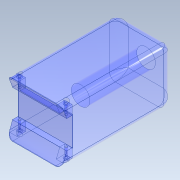
# Autodesk Inventor part: shank_front_v2
Saved by Autodesk Inventor 2020 (Build 240168000, 168)
## iProperties
Created: 2021-01-30
Part Number: shank_front_v2
Material: Generic
Document SubType Name: Modeling
Designer: DELL
Density: 1 g/cm^3
Appearance: Clear - Blue
Mass: 1058.53 g
Surface Area: 891.515 cm^2
Volume: 1058.53 cm^3
Author: DELL
Autodesk Inventor part; units mm, degrees
ref_plane "YZ Plane" through (0, 0, 0) normal (1, 0, 0) x (0, 1, 0)
ref_plane "XY Plane" through (0, 0, 0) normal (0, 0, 1) x (1, 0, 0)
ref_plane "UCS1: YZ Plane" through (0, 0, 0) normal (1, 0, 0) x (0, 1, 0)
sketch "Sketch16" plane through (0, 0, 0) normal (1, 0, 0) x (0, 1, 0)
  circle A0 centre (0, 0) radius 56
  line L0 (0, -212.6874) -> (0, 100.7812) construction
  line L1 (-29, -60) -> (29, -60)
  line L2 (-15, -53.9537) -> (-15, -60)
  line L3 (-6, -55.6776) -> (-6, -60)
  line L4 (6, -55.6776) -> (6, -60)
  line L5 (15, -53.9537) -> (15, -60)
  line L6 (29, -47.9062) -> (29, -167.9062)
  line L7 (29, -167.9062) -> (-29, -167.9062)
  line L8 (-29, -167.9062) -> (-29, -47.9062)
  dimension "d156" = 112
  dimension "d183" = 60
  dimension "d184" = 12
  dimension "d185" = 30
  dimension "d209" = 58
  dimension "d210" = 120
  constraints: 16 end point, 6 perpendicular, 6 point on circle, 6 point on line, 1 centre point, 1 coincident, 1 horizontal, 1 vertical, 3 other
  measures "d156" diameter of A0
  measures "d183" distance from line of point (0, 0) L1
  measures "d184" distance between parallel lines of L4 L3
  measures "d185" distance between parallel lines of L5 L2
  measures "d209" distance of L6.end L7.end
  measures "d210" distance of L7.end L8.end
extrude "Extrusion14" add sketch "Sketch16" along normal mid plane 58 contours A0 L2 L1 L8 | L6 L1 L5 A0 | L1 L6 L7 L8
fillet "Fillet12" radius 6 4 edges at (-29, 29, -107.9062) (-29, -29, -107.9062) (29, -29, -107.9062) (29, 29, -107.9062)
sketch "Sketch20" plane through (0, 0, 0) normal (0, 1, 0) x (-1, 0, 0)
  circle A0 centre (-25, -57.5) radius 1.25
  circle A1 centre (25, -57.5) radius 1.25
  circle A2 centre (-25, -57.5) radius 2.5
  circle A3 centre (25, -57.5) radius 2.5
  line L0 (-29, -60) -> (29, -60) projected
  line L1 (0, -47.9062) -> (0, -60) construction
  line L2 (23, -47.9062) -> (-23, -47.9062) construction
  point P0 (0, 0)
  dimension "d192" = 2.5
  dimension "d193" = 5
  dimension "d194" = 50
  dimension "d195" = 2.5
  constraints: 4 centre point, 2 coincident, 2 end point, 2 equal radius, 2 midpoint, 1 horizontal alignment, 1 symmetric about line
  measures "d192" diameter of A0
  measures "d193" diameter of A2
  measures "d194" distance of A1.centre A0.centre
  measures "d195" distance from line of L0 A0.centre
extrude "Extrusion17" cut sketch "Sketch20" against normal through all both and the other way through all contours A0 | A1
ref_plane "Work Plane6" through (0, 29.5, 0) normal (0, 1, 0) x (-1, 0, 0)
ref_plane "Work Plane7" through (0, -29.5, 0) normal (0, 1, 0) x (-1, 0, 0)
sketch "Sketch21" plane through (0, 0, 0) normal (0, 1, 0) x (-1, 0, 0)
  circle A0 centre (-25, -57.5) radius 1.25 projected
  circle A1 centre (-25, -57.5) radius 2.5
  circle A2 centre (25, -57.5) radius 1.25 projected
  circle A3 centre (25, -57.5) radius 2.5
  point P0 (0, 0)
  dimension "d200" = 5
  constraints: 2 centre point, 2 coincident, 1 equal radius
  measures "d200" diameter of A1
extrude "Extrusion18" cut sketch "Sketch21" against normal blind 4.5 from surface at 29.5 contours A0 | A1 | A2 | A3
extrude "Extrusion19" cut sketch "Sketch21" along normal blind 4.5 from surface at -29.5 contours A0 | A1 | A2 | A3
sketch "Sketch22" plane through (-29, 15, -60) normal (0, 0, 1) x (1, 0, 0)
  line L0 (29, -15) -> (29, 14) construction
  line L1 (0, 8.0076) -> (0, 0)
  line L2 (8, 14) -> (0, 14)
  line L3 (0, 14) -> (0, 0)
  line L4 (0, 0) -> (8, 0)
  line L5 (8, 0) -> (8, 14)
  line L6 (0, -30) -> (0, 0) projected
  line L7 (6, 14) -> (52, 14) projected
  line L8 (0, 0) -> (58, 0) projected
  line L9 (29, -15) -> (58, -15) construction
  line L10 (58, 0) -> (50, 0)
  line L11 (58, 14) -> (58, 0)
  line L12 (50, 14) -> (58, 14)
  line L13 (50, 0) -> (50, 14)
  line L14 (0, -44) -> (0, -30)
  line L15 (8, -44) -> (0, -44)
  line L16 (8, -30) -> (8, -44)
  line L17 (0, -30) -> (58, -30)
  line L18 (50, -30) -> (50, -44)
  line L19 (50, -44) -> (58, -44)
  line L20 (58, -44) -> (58, -30)
  line L21 (8, 10) -> (0, 10)
  line L22 (1.5, 10) -> (6.5, 10) projected
  line L23 (56.5, 10) -> (51.5, 10)
  line L24 (50, 10) -> (58, 10)
  line L25 (8, -40) -> (0, -40)
  line L26 (50, -40) -> (58, -40)
  point P0 (29, -15)
  point P1 (6, -44)
  point P2 (8, -40)
  point P3 (58, 10)
  dimension "d211" = 8
  constraints: 46 end point, 19 symmetric about line, 5 collinear, 2 point on line, 1 coincident, 1 horizontal, 1 midpoint, 1 perpendicular, 1 vertical
  measures "d211" distance between parallel lines of L3 L5
thicken "Thicken1" operation new thickness 0.6 both sides no extend neighbours no toward (0, -0.483449, -0.8753725) faces at (7.755, -27.0731, -49.0209) (8.1856, -15, -54.7462) (9.6667, -5, -60) (8.1856, 15, -54.7462) (7.6667, 27.1275, -48.9908)
extrude "Extrusion20" add sketch "Sketch22" along normal blind 15 separate body contours L3 L21 L5 L4 L1 | L13 L24 L23 L11 L8 | L14 L17 L16 L25 | L17 L20 L26 L18
combine bodies "Combine1" operation type add bodies to combine 3 2
combine bodies "Combine2" operation type common bodies to combine 3 1 keep tools yes
fillet "Fillet13" radius 10 8 edges at (-27.2426, -27.2426, -167.9062) (0, -29, -167.9062) (27.2426, -27.2426, -167.9062) (29, 0, -167.9062) (27.2426, 27.2426, -167.9062) (0, 29, -167.9062) (-27.2426, 27.2426, -167.9062) (-29, 0, -167.9062)
sketch "Sketch23" plane through (19, 19, -167.9062) normal (0, 0, -1) x (-1, 0, 0)
  circle A0 centre (19, -19) radius 10
  dimension "d213" = 20
  constraints: 1 centre point, 1 coincident
  measures "d213" diameter of A0
extrude "Extrusion21" cut sketch "Sketch23" against normal blind 70 bodies 1
body "Solid1"
body "Solid6"
body "Solid9"
